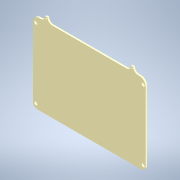
# Autodesk Inventor part: back plate
Saved by Autodesk Inventor 2022 (Build 260153000, 153)
## iProperties
Created: 2021-05-28
Part Number: back plate
Material: Nylon 6/6
Document SubType Name: Modeling
Designer: benka
Density: 1.13 g/cm^3
Appearance: Nylon 6
Author: benka
Autodesk Inventor part; units mm, degrees
ref_plane "YZ Plane" through (0, 0, 0) normal (1, 0, 0) x (0, 1, 0)
ref_plane "XZ Plane" through (0, 0, 0) normal (0, 1, 0) x (-1, 0, 0)
ref_plane "XY Plane" through (0, 0, 0) normal (0, 0, 1) x (1, 0, 0)
sketch "Sketch1" plane through (0, 0, 0) normal (0, 0, 1) x (1, 0, 0)
  ellipse E0 centre (-218.5917, 142.4744) end of major axis (-220.586, 142.4744) minor radius 1.993
  ellipse E1 centre (55.7593, 142.4744) end of major axis (53.765, 142.4744) minor radius 1.993
  line L0 (-222.6278, 147.4744) -> (-215.1278, 147.4744)
  line L1 (52.1593, 147.4744) -> (59.6593, 147.4744)
  line L2 (99.1593, 127.7477) -> (99.1593, -118.8668)
  line L3 (-262.1278, 127.7477) -> (-262.1278, -118.8668)
  line L4 (-257.1278, -123.8668) -> (94.1593, -123.8668)
  line L5 (94.1593, 132.7477) -> (74.1593, 132.7477)
  line L6 (59.6593, 147.2477) -> (59.6593, 147.4744)
  line L7 (52.1593, 147.4744) -> (52.1593, 147.2477)
  line L8 (-215.1278, 147.2477) -> (-215.1278, 147.4744)
  line L9 (-222.6278, 147.4744) -> (-222.6278, 147.2477)
  line L10 (-237.1278, 132.7477) -> (-257.1278, 132.7477)
  arc A0 (59.6593, 147.2477) -> (74.1593, 132.7477) centre (74.1593, 147.2477) ccw
  arc A1 (37.6593, 132.7477) -> (52.1593, 147.2477) centre (37.6593, 147.2477) ccw
  arc A2 (-215.1278, 147.2477) -> (-200.6278, 132.7477) centre (-200.6278, 147.2477) ccw
  arc A3 (-237.1278, 132.7477) -> (-222.6278, 147.2477) centre (-237.1278, 147.2477) ccw
  line L11 (37.6593, 132.7477) -> (-200.6278, 132.7477)
  arc A4 (94.1593, -123.8668) -> (99.1593, -118.8668) centre (94.1593, -118.8668) ccw
  arc A5 (-262.1278, -118.8668) -> (-257.1278, -123.8668) centre (-257.1278, -118.8668) ccw
  arc A6 (-257.1278, 132.7477) -> (-262.1278, 127.7477) centre (-257.1278, 127.7477) ccw
  arc A7 (99.1593, 127.7477) -> (94.1593, 132.7477) centre (94.1593, 127.7477) ccw
  circle A8 centre (90.6553, 119.8422) radius 5
  circle A9 centre (90.6553, -115.1578) radius 5
  circle A10 centre (-253.3447, -115.1578) radius 5
  circle A11 centre (-253.3447, 119.8422) radius 5
  point P0 (-262.1278, -108.8668)
  point P1 (-247.1278, -123.8668)
  point P2 (-262.1278, 112.7477)
  point P3 (99.1593, 112.7477)
  point P4 (59.6593, 132.7477)
  point P5 (-222.6278, 132.7477)
  point P6 (-242.1278, 132.7477)
  point P7 (79.1593, 132.7477)
  point P8 (59.6593, 147.361)
  point P9 (84.1593, -123.8668)
  point P10 (99.1593, -108.8668)
  dimension "d3" = 7.5
  dimension "d4" = 7.5
  dimension "d18" = 5
  dimension "d28" = 14.7267
  dimension "d29" = 14.5
  dimension "d33" = 5
  dimension "d34" = 4.7733
  dimension "d36" = 5
  dimension "d37" = 5
  dimension "d39" = 5
  constraints: 24 end point, 16 point on circle, 14 tangent, 12 centre point, 12 point on line, 6 equal radius, 2 horizontal, 1 collinear, 1 midpoint, 1 parallel, 1 perpendicular, 1 vertical, 12 other
  measures "d3" distance of L0.start L0.end
  measures "d4" distance of L1.end L1.start
  measures "d18" distance from line of L1 point (55.759, 142.474)
  measures "d28" distance of point (59.659, 132.748) L1.end
  measures "d29" radius of A0
  measures "d33" distance from line of L0 point (-218.592, 142.474)
  measures "d34" vertical distance of L8.start point (-218.592, 142.474)
  measures "d36" distance of L10.start point (-242.128, 132.748)
  measures "d37" distance of point (79.159, 132.748) L5.end
  measures "d39" radius of A4
extrude "Extrusion1" add sketch "Sketch1" along normal blind 5
body "Solid1"
